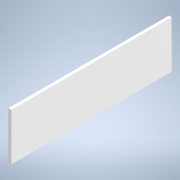
# Autodesk Inventor part: backPlate
Saved by Autodesk Inventor 2021.2 (Build 252289000, 289)
## iProperties
Created: 2021-02-12
Part Number: backPlate
Material: PC/ABS Plastic
Document SubType Name: Modeling
Designer: robst
Density: 0.357273 g/cm^3
Appearance: Smooth - White
Author: robst
Autodesk Inventor part; units mm, degrees
ref_plane "YZ Plane" through (0, 0, 0) normal (1, 0, 0) x (0, 1, 0)
ref_plane "XZ Plane" through (0, 0, 0) normal (0, 1, 0) x (-1, 0, 0)
ref_plane "XY Plane" through (0, 0, 0) normal (0, 0, 1) x (1, 0, 0)
sketch "Sketch1" plane through (0, 0, 0) normal (1, 0, 0) x (0, 1, 0)
  line L0 (-9.525, 53.975) -> (-9.525, -53.975)
  line L1 (-9.525, -53.975) -> (9.525, -53.975)
  line L2 (9.525, -53.975) -> (9.525, 53.975)
  line L3 (9.525, 53.975) -> (-9.525, 53.975)
  line L4 (-9.525, 53.975) -> (9.525, -53.975) construction
  line L5 (-9.525, -53.975) -> (9.525, 53.975) construction
  point P0 (0, 0)
  dimension "d2" = 19.05
  dimension "d3" = 107.95
  constraints: 12 end point, 2 midpoint, 2 parallel, 1 perpendicular, 1 vertical
  measures "d2" distance between parallel lines of L2 L0
  measures "d3" distance between parallel lines of L1 L3
extrude "Extrusion1" add sketch "Sketch1" against normal blind 1.905
body "Solid1"
